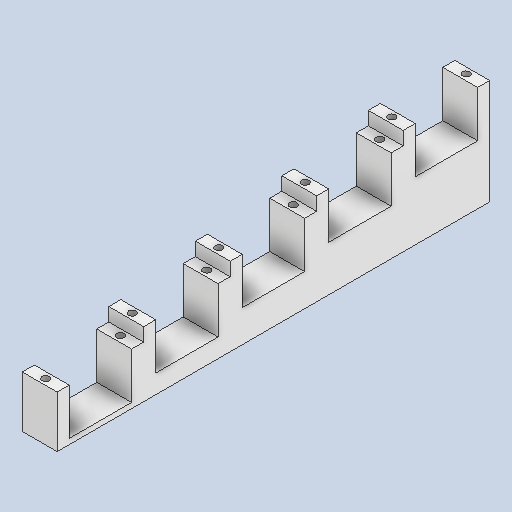
# Autodesk Inventor part: Forearm_1
Saved by Autodesk Inventor 2022 (Build 260153000, 153)
## iProperties
Created: 2023-01-15
Part Number: Forearm_1
Material: ABS Plastic
Document SubType Name: Modeling
Designer: 48735
Density: 1.06 g/cm^3
Appearance: Smooth - White
Author: 48735
Autodesk Inventor part; units mm, degrees
ref_plane "YZ Plane" through (0, 0, 0) normal (1, 0, 0) x (0, 1, 0)
ref_plane "XZ Plane" through (0, 0, 0) normal (0, 1, 0) x (-1, 0, 0)
sketch "Sketch15" plane through (0, 0, 0) normal (0, 1, 0) x (-1, 0, 0)
  line L0 (0, 0) -> (-13, 0)
  line L1 (-13, 0) -> (-13, 160)
  line L2 (-13, 160) -> (0, 160)
  line L3 (0, 160) -> (0, 0)
  line L4 (-13, 0) -> (-13, -1.5)
  line L5 (-13, -1.5) -> (0, -1.5)
  line L6 (0, -1.5) -> (0, 0)
  dimension "d75" = 13
  dimension "d76" = 160
  dimension "d127" = 1.5
  constraints: 14 end point, 3 perpendicular, 2 parallel, 1 horizontal, 1 vertical
  measures "d75" distance of L1.end L2.end
  measures "d76" distance of L0.end L1.end
  measures "d127" distance of L0.end L4.end
extrude "Extrusion15" add sketch "Sketch15" along normal blind 2
sketch "Sketch16" plane through (0, 2, 0) normal (0, 1, 0) x (1, 0, 0)
  line L0 (0, 0) -> (0, -160) projected
  line L1 (13, -160) -> (13, 1.5) projected
  line L2 (0, -160) -> (13, -160)
  line L3 (13, -160) -> (13, -155.5)
  line L4 (13, -155.5) -> (0, -155.5)
  line L5 (0, -155.5) -> (0, -160)
  circle A0 centre (6.5, -157.75) radius 1.4
  circle A1 centre (6.5, -129.95) radius 1.4
  line L6 (13, -127.7) -> (13, -132.2)
  line L7 (13, -132.2) -> (0, -132.2)
  line L8 (0, -127.7) -> (13, -127.7)
  line L9 (0, -127.7) -> (0, -132.2)
  point P0 (20, 0)
  point P1 (13, -160)
  point P2 (0, -155.5)
  point P3 (13, 1.5)
  constraints: 16 end point, 3 perpendicular, 2 centre point, 2 parallel, 2 point on line, 1 collinear, 1 horizontal, 4 other
extrude "Extrusion16" add sketch "Sketch16" along normal blind 17.25 contours L8 L1 L7 L0 | L4 L1 L2 L0 | A0 | A1
sketch "Sketch20" plane through (0, 2, 0) normal (0, 1, 0) x (1, 0, 0)
  line L0 (0, -127.7) -> (13, -127.7) projected
  line L1 (0, -127.7) -> (0, -123.2)
  line L2 (0, 0) -> (0, -127.7) projected
  line L3 (0, -123.2) -> (13, -123.2)
  line L4 (13, -127.7) -> (13, 1.5) projected
  line L5 (13, -127.7) -> (13, -123.2)
  line L6 (13, -132.2) -> (13, -127.7) projected
  line L7 (13, -127.7) -> (0, -127.7)
  circle A0 centre (6.5, -125.45) radius 1.4
  circle A1 centre (6.5, -97.65) radius 1.4
  line L8 (10, -95.4) -> (13, -95.4)
  line L9 (13, -95.4) -> (13, -99.9)
  line L10 (13, -99.9) -> (0, -99.9)
  line L11 (0, -95.4) -> (10, -95.4)
  line L12 (0, -95.4) -> (0, -99.9)
  line L13 (6.5, -123.2) -> (6.5, -125.45)
  point P0 (20, 0)
  point P1 (13, 1.5)
  dimension "d95" = 4.5
  dimension "d96" = 2.8
  constraints: 20 end point, 4 perpendicular, 4 point on line, 2 centre point, 2 collinear, 1 horizontal, 1 midpoint, 1 vertical, 4 other
  measures "d95" distance of L0.start L1.end
  measures "d96" diameter of A0
extrude "Extrusion20" add sketch "Sketch20" along normal blind 22.25 contours A0 | L1 L3 L4 L0 | L2 L11 L8 L4 L10 | A1
sketch "Sketch21" plane through (0, 2, 0) normal (0, 1, 0) x (1, 0, 0)
  line L0 (13, -95.4) -> (0, -95.4) projected
  line L1 (0, -95.4) -> (0, -90.9)
  line L2 (0, 0) -> (0, -160) projected
  line L3 (13, -160) -> (13, 1.5) projected
  line L4 (0, -95.4) -> (13, -95.4)
  circle A0 centre (6.5, -93.15) radius 1.4
  circle A1 centre (6.5, -65.35) radius 1.4
  line L5 (10, -63.1) -> (13, -63.1)
  line L6 (13, -63.1) -> (13, -67.6)
  line L7 (13, -67.6) -> (0, -67.6)
  line L8 (0, -67.6) -> (0, -63.1)
  line L9 (0, -63.1) -> (10, -63.1)
  line L10 (13, -95.4) -> (13, -90.9)
  line L11 (0, -90.9) -> (13, -90.9)
  point P0 (20, -90.9)
  point P1 (20, 0)
  point P2 (13, 1.5)
  dimension "d102" = 4.5
  constraints: 18 end point, 4 point on line, 2 centre point, 2 collinear, 2 perpendicular, 1 horizontal, 4 other
  measures "d102" distance of L0.end L1.end
extrude "Extrusion21" add sketch "Sketch21" along normal blind 27.25 contours L0 L1 L11 L3 | L7 L2 L9 L5 L3 | A0 | A1
sketch "Sketch22" plane through (0, 2, 0) normal (0, 1, 0) x (1, 0, 0)
  line L0 (0, -63.1) -> (13, -63.1) projected
  line L1 (0, -63.1) -> (0, -58.6)
  line L2 (0, 0) -> (0, -160) projected
  line L3 (0, -58.6) -> (13, -58.6)
  line L4 (13, -160) -> (13, 1.5) projected
  line L5 (13, -58.6) -> (13, -63.1)
  line L6 (13, -63.1) -> (0, -63.1)
  circle A0 centre (6.5, -60.85) radius 1.4
  circle A1 centre (6.5, -33.05) radius 1.4
  line L7 (10, -30.8) -> (13, -30.8)
  line L8 (13, -30.8) -> (13, -35.3)
  line L9 (13, -35.3) -> (0, -35.3)
  line L10 (0, -30.8) -> (0, -35.3)
  line L11 (0, -30.8) -> (10, -30.8)
  line L12 (6.5, -58.6) -> (6.5, -60.85)
  point P0 (20, 0)
  point P1 (13, 1.5)
  dimension "d110" = 4.5
  dimension "d111" = 2.8
  constraints: 20 end point, 4 perpendicular, 3 point on line, 2 centre point, 2 vertical, 1 collinear, 1 horizontal, 1 midpoint, 4 other
  measures "d110" distance of L0.start L1.end
  measures "d111" diameter of A0
extrude "Extrusion22" add sketch "Sketch22" along normal blind 32.25 contours A0 | L1 L3 L4 L0 | L2 L11 L7 L4 L9 | A1
sketch "Sketch23" plane through (0, 2, 0) normal (0, 1, 0) x (1, 0, 0)
  line L0 (0, -30.8) -> (13, -30.8) projected
  line L1 (0, -30.8) -> (0, -26.3)
  line L2 (0, 0) -> (0, -160) projected
  line L3 (0, -26.3) -> (13, -26.3)
  line L4 (13, -160) -> (13, 1.5) projected
  line L5 (13, -26.3) -> (13, -30.8)
  line L6 (13, -30.8) -> (0, -30.8)
  circle A0 centre (6.5, -28.55) radius 1.4
  circle A1 centre (6.5, -0.75) radius 1.4
  line L7 (20, 0) -> (0, 0) projected
  line L8 (3, 1.5) -> (13, 1.5)
  line L9 (13, 1.5) -> (13, -3)
  line L10 (13, -3) -> (0, -3)
  line L11 (0, -3) -> (0, 1.5)
  line L12 (0, 1.5) -> (3, 1.5)
  line L13 (6.5, -26.3) -> (6.5, -28.55)
  dimension "d118" = 4.5
  dimension "d119" = 2.8
  dimension "d124" = 4.5
  constraints: 20 end point, 5 perpendicular, 3 point on line, 2 centre point, 2 vertical, 1 midpoint, 3 other
  measures "d118" distance of L0.start L1.end
  measures "d119" diameter of A0
  measures "d124" distance of L8.end L9.end
extrude "Extrusion23" add sketch "Sketch23" along normal blind 37.25 contours A0 | L1 L3 L4 L0 | L2 L7 A1 L4 L10 | L11 L12 L8 L4 L7 A1 | L7 A1 | A1 L7
sketch "Sketch27" plane through (0, 2, 0) normal (0, 1, 0) x (1, 0, 0)
  line L0 (0, -123.2) -> (13, -123.2) projected
  line L1 (0, -99.9) -> (13, -99.9) projected
  line L2 (0, -123.2) -> (13, -123.2)
  line L3 (13, -123.2) -> (13, -99.9)
  line L4 (13, -99.9) -> (0, -99.9)
  line L5 (0, -99.9) -> (0, -123.2)
  point P0 (0, 0)
  constraints: 8 end point, 2 parallel, 1 horizontal, 1 perpendicular
extrude "Extrusion27" add sketch "Sketch27" along normal blind 5
sketch "Sketch28" plane through (0, 2, 0) normal (0, 1, 0) x (1, 0, 0)
  line L0 (13, -90.9) -> (13, -67.6) projected
  line L1 (0, -67.6) -> (0, -90.9) projected
  line L2 (13, -90.9) -> (0, -90.9)
  line L3 (0, -90.9) -> (0, -67.6)
  line L4 (0, -67.6) -> (13, -67.6)
  line L5 (13, -67.6) -> (13, -90.9)
  point P0 (0, 0)
  constraints: 8 end point, 2 parallel, 1 horizontal, 1 perpendicular
extrude "Extrusion28" add sketch "Sketch28" along normal blind 10
sketch "Sketch29" plane through (0, 2, 0) normal (0, 1, 0) x (1, 0, 0)
  line L0 (13, -58.6) -> (0, -58.6) projected
  line L1 (0, -58.6) -> (13, -58.6)
  line L2 (13, -58.6) -> (13, -35.3)
  line L3 (13, -35.3) -> (0, -35.3)
  line L4 (0, -35.3) -> (0, -58.6)
  point P0 (0, 0)
  constraints: 8 end point, 2 parallel, 1 horizontal, 1 perpendicular
extrude "Extrusion29" add sketch "Sketch29" along normal blind 15
sketch "Sketch30" plane through (0, 2, 0) normal (0, 1, 0) x (1, 0, 0)
  line L0 (0, -26.3) -> (13, -26.3) projected
  line L1 (0, -3) -> (13, -3) projected
  line L2 (0, -26.3) -> (13, -26.3)
  line L3 (13, -26.3) -> (13, -3)
  line L4 (13, -3) -> (0, -3)
  line L5 (0, -3) -> (0, -26.3)
  point P0 (0, 0)
  constraints: 8 end point, 2 parallel, 1 horizontal, 1 perpendicular
extrude "Extrusion30" add sketch "Sketch30" along normal blind 20
ref_plane "Work Plane1" through (0, 0, -1.5) normal (0, 0, 1) x (1, 0, 0)
ref_plane "Work Plane4" through (0, 0, 30.8) normal (0, 0, 1) x (1, 0, 0)
ref_plane "Work Plane3" through (0, 0, 95.4) normal (0, 0, 1) x (1, 0, 0)
sketch "Sketch35" plane through (0, 19.25, 0) normal (0, 1, 0) x (1, 0, 0)
  line L0 (0, -160) -> (13, -160) projected
  line L1 (6.5, -160) -> (6.5, -157.75)
  line L2 (6.5, -157.75) -> (6.5, -129.95)
  point P0 (0, 0)
  dimension "d168" = 2.25
  dimension "d169" = 27.8
  constraints: 4 end point, 1 midpoint, 1 point on line, 1 vertical
  measures "d168" distance of L1.start L1.end
  measures "d169" distance of L1.end L2.end
hole "Hole1" at (6.5, 19.25, 129.95) at (6.5, 19.25, 157.75) direction (0, -1, 0) diameter 2.8 depth 3
sketch "Sketch36" plane through (0, 24.25, 0) normal (0, 1, 0) x (1, 0, 0)
  line L0 (0, -127.7) -> (13, -127.7) projected
  line L1 (6.5, -127.7) -> (6.5, -125.45)
  line L2 (6.5, -125.45) -> (6.5, -97.65)
  point P0 (0, 0)
  constraints: 4 end point, 1 midpoint, 1 point on line, 1 vertical
hole "Hole2" at (6.5, 24.25, 125.45) at (6.5, 24.25, 97.65) direction (0, -1, 0) diameter 2.8 depth 3
sketch "Sketch37" plane through (0, 29.25, 0) normal (0, 1, 0) x (1, 0, 0)
  line L0 (0, -95.4) -> (13, -95.4) projected
  line L1 (6.5, -95.4) -> (6.5, -93.15)
  line L2 (6.5, -93.15) -> (6.5, -65.35)
  point P0 (0, 0)
  constraints: 4 end point, 1 midpoint, 1 point on line, 1 vertical
hole "Hole3" at (6.5, 29.25, 93.15) at (6.5, 29.25, 65.35) direction (0, -1, 0) diameter 2.8 depth 3
sketch "Sketch38" plane through (0, 34.25, 0) normal (0, 1, 0) x (1, 0, 0)
  line L0 (0, -63.1) -> (13, -63.1) projected
  line L1 (6.5, -63.1) -> (6.5, -60.85)
  line L2 (6.5, -60.85) -> (6.5, -33.05)
  point P0 (0, 0)
  dimension "d195" = 2.25
  dimension "d196" = 27.8
  constraints: 4 end point, 1 midpoint, 1 point on line, 1 vertical
  measures "d195" distance of L1.start L1.end
  measures "d196" distance of L1.end L2.end
hole "Hole4" at (6.5, 34.25, 60.85) at (6.5, 34.25, 33.05) direction (0, -1, 0) diameter 2.8 depth 3
sketch "Sketch39" plane through (0, 39.25, 0) normal (0, 1, 0) x (1, 0, 0)
  line L0 (13, -30.8) -> (0, -30.8) projected
  line L1 (6.5, -30.8) -> (6.5, -28.55)
  line L2 (6.5, -28.55) -> (6.5, -0.75)
  point P0 (0, 0)
  dimension "d204" = 2.25
  dimension "d205" = 27.8
  constraints: 4 end point, 1 midpoint, 1 point on line, 1 vertical
  measures "d204" distance of L1.start L1.end
  measures "d205" distance of L1.end L2.end
hole "Hole5" at (6.5, 39.25, 28.55) at (6.5, 39.25, 0.75) direction (0, -1, 0) diameter 2.8 depth 3
thread "Thread1" size "M3x0.5" class "6H" standard "ANSI Metric M Profile" length 6
thread "Thread2" size "M3x0.5" class "6H" standard "ANSI Metric M Profile" length 6
thread "Thread3" size "M3x0.5" class "6H" standard "ANSI Metric M Profile" length 6
thread "Thread4" size "M3x0.5" class "6H" standard "ANSI Metric M Profile" length 6
thread "Thread5" size "M3x0.5" class "6H" standard "ANSI Metric M Profile" length 6
thread "Thread6" size "M3x0.5" class "6H" standard "ANSI Metric M Profile" length 6
thread "Thread7" size "M3x0.5" class "6H" standard "ANSI Metric M Profile" length 6
thread "Thread8" size "M3x0.5" class "6H" standard "ANSI Metric M Profile" length 6
thread "Thread9" size "M3x0.5" class "6H" standard "ANSI Metric M Profile" length 6
thread "Thread10" size "M3x0.5" class "6H" standard "ANSI Metric M Profile" length 6
ref_plane "Work Plane2" through (0, 0, 160) normal (0, 0, 1) x (1, 0, 0)
body "Solid2"
